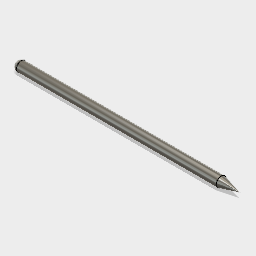
铅笔 v1 (Autodesk Fusion 360 design; units mm, degrees)
Autodesk Fusion 360 part; units mm, degrees
cylinder "圆柱体基本要素1" add diameter 2 height 40 placed x (0, 0, -1) y (0, 1, 0) z (1, 0, 0) at (0, 0, 0)
sphere "球体基本要素1" cut diameter 2 placed x (0, 0, -1) y (0, 1, 0) z (1, 0, 0) at (0, 0, 0)
sphere "球体基本要素2" add diameter 2 placed x (0, 0, -1) y (0, 1, 0) z (1, 0, 0) at (0, 0, 0)
extrude "拉伸1" add 1 faces at (40, 0.5031, 0.3296) along direction (1, 0, 0) blind 3.7 draft -15
